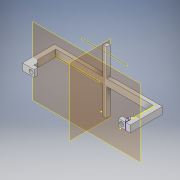
# Autodesk Inventor part: tec_holder_part2
Saved by Autodesk Inventor 2018 (Build 220112000, 112)
## iProperties
Created: 2018-02-10
Part Number: tec_holder_part2
Material: Generic
Document SubType Name: Modeling
Designer: Benedikt
Density: 1 g/cm^3
Appearance: Default
Author: Benedikt
## iProperties of the stored document tec_holder_part2_3DPrint.ipt
Created: 2018-02-10
Part Number: tec_holder_part2_3DPrint
Material: Generic
Document SubType Name: Modeling
Designer: Benedikt
Density: 1 g/cm^3
Appearance: Default
Author: Benedikt
Autodesk Inventor part; units mm, degrees
ref_plane "YZ Plane" through (0, 0, 0) normal (1, 0, 0) x (0, 1, 0)
ref_plane "XZ Plane" through (0, 0, 0) normal (0, 1, 0) x (-1, 0, 0)
ref_plane "XY Plane" through (0, 0, 0) normal (0, 0, 1) x (1, 0, 0)
ref_plane "Work Plane1" through (-37.0541, 3.9333, 19.6842) normal (0, 1, 0) x (-1, 0, 0)
sketch "Sketch1" plane through (-37.0541, 3.9333, 19.6842) normal (0, 1, 0) x (-1, 0, 0)
  point P0 (-37.0541, -19.6842)
ref_plane "Work Plane2" through (-37.0541, 26.9333, 19.6842) normal (0, 1, 0) x (-1, 0, 0)
sketch "Sketch2" plane through (-37.0541, 26.9333, 19.6842) normal (0, 1, 0) x (-1, 0, 0)
  line L0 (-16.9, -6.2922) -> (-16.9, -34.5181) construction
  line L1 (-18.4, -45.1) -> (-15.4, -45.1)
  line L2 (-15.4, 4.9) -> (-18.4, 4.9)
  line L3 (-15.4, -45.1) -> (-16.9, -20.1) construction
  line L4 (-17.065, -17.35) -> (-18.4, 4.9) construction
  line L5 (26.6, -17.35) -> (-15.4, -17.35)
  line L6 (-16.735, -17.35) -> (-17.065, -17.35)
  line L7 (-18.4, -17.35) -> (-60.4, -17.35)
  line L8 (-18.4, 4.9) -> (-18.4, -17.35)
  line L9 (-18.4, -22.85) -> (-18.4, -45.1)
  line L10 (-15.4, -45.1) -> (-15.4, -22.85)
  line L11 (-15.4, -17.35) -> (-15.4, 4.9)
  line L12 (-15.4, -22.85) -> (26.6, -22.85)
  line L13 (-18.4, -45.1) -> (-17.065, -22.85) construction
  line L14 (-16.9, -20.1) -> (-15.4, 4.9) construction
  line L15 (-60.4, -22.85) -> (-18.4, -22.85)
  line L16 (-17.065, -22.85) -> (-16.735, -22.85)
  line L17 (-60.4, -17.35) -> (-60.4, -22.85)
  line L18 (26.6, -17.35) -> (26.6, -22.85)
  point P0 (-37.0541, -19.6842)
  point P1 (22.6, -17.35)
  point P2 (-56.4, -22.85)
  dimension "d3" = 3
  dimension "d4" = 50
  dimension "d5" = 42
  dimension "d6" = 42
  constraints: 38 end point, 14 parallel, 4 horizontal, 3 perpendicular, 3 point on line, 2 vertical, 2 other
  measures "d3" distance of L2.end L2.start
  measures "d4" distance of L2.start L1.end
  measures "d5" distance between parallel lines of L9 L17
  measures "d6" distance between parallel lines of L18 L10
extrude "Extrusion2" add sketch "Sketch2" along normal blind 3
sketch "Sketch3" plane through (-37.0541, 26.9333, 19.6842) normal (0, -1, 0) x (1, 0, 0)
  line L0 (60.4, -22.85) -> (18.4, -22.85) projected
  line L1 (18.4, -17.35) -> (60.4, -17.35) projected
  line L2 (60.4, -22.85) -> (56.4, -22.85)
  line L3 (56.4, -22.85) -> (56.4, -17.35)
  line L4 (56.4, -17.35) -> (60.4, -17.35)
  line L5 (60.4, -17.35) -> (60.4, -22.85)
  line L6 (-26.6, -22.85) -> (-26.6, -17.35) projected
  line L7 (-26.6, -17.35) -> (15.4, -17.35) projected
  line L8 (-26.6, -22.85) -> (-22.6, -22.85)
  line L9 (-22.6, -22.85) -> (-22.6, -17.35)
  line L10 (-22.6, -17.35) -> (-26.6, -17.35)
  line L11 (-26.6, -17.35) -> (-26.6, -22.85)
  point P0 (37.0541, -19.6842)
  dimension "d9" = 4
  dimension "d10" = 4
  constraints: 16 end point, 4 parallel, 2 horizontal, 2 perpendicular, 2 point on line
  measures "d9" distance of L3.end L4.end
  measures "d10" distance of L10.end L9.end
extrude "Extrusion3" add sketch "Sketch3" along normal blind 23
sketch "Sketch4" plane through (19.3459, 26.9333, -3.1658) normal (-1, 0, 0) x (0, 0, 1)
  line L0 (5.5, -23) -> (0, -23) projected
  line L1 (5.5, 0) -> (5.5, -23) projected
  line L2 (0, -23) -> (5.5, -23)
  line L3 (5.5, -23) -> (5.5, -19)
  line L4 (5.5, -19) -> (0, -19)
  line L5 (0, -19) -> (0, -23)
  point P0 (3.1658, -26.9333)
  dimension "d13" = 4
  constraints: 8 end point, 2 parallel, 1 horizontal, 1 perpendicular, 1 point on line
  measures "d13" distance of L3.end L2.end
sketch "Sketch5" plane through (-18.6541, 29.9333, 2.3342) normal (0, 0, 1) x (1, 0, 0)
  line L0 (38, -3) -> (38, -26) projected
  line L1 (38, -26) -> (32.5, -26)
  line L2 (32.5, -26) -> (32.5, -23)
  line L3 (32.5, -23) -> (38, -17.8732)
  point P0 (18.6541, -29.9333)
  dimension "d14" = 5.5
  dimension "d15" = 3
  constraints: 6 end point, 1 horizontal, 1 perpendicular, 1 point on line
  measures "d14" distance of L0.end L1.end
  measures "d15" distance of L1.end L2.end
extrude "Extrusion4" add sketch "Sketch5" against normal up to surface (5.5 mm away)
ref_plane "Work Plane3" through (-20.1541, 26.9333, 2.3342) normal (1, 0, 0) x (0, 0, -1)
mirror "Mirror1" about plane through (-20.1541, 26.9333, 2.3342) normal (1, 0, 0) of "Extrusion4"
ref_plane "Work Plane4" through (-37.0541, 12.1833, 19.6842) normal (0, -1, 0) x (1, 0, 0)
sketch "Sketch6" plane through (-37.0541, 12.1833, 19.6842) normal (0, -1, 0) x (1, 0, 0)
  circle A0 centre (53.4, -20.1) radius 1.7 projected
  circle A1 centre (-19.6, -20.1) radius 1.7 projected
  line L0 (-16.8355, -21.7765) -> (-19.6696, -23.3324)
  line L1 (-19.6696, -23.3324) -> (-22.4342, -21.6559)
  line L2 (-22.4342, -21.6559) -> (-22.3645, -18.4234)
  line L3 (-22.3645, -18.4234) -> (-19.5303, -16.8676)
  line L4 (-19.5303, -16.8676) -> (-16.7658, -18.5441)
  line L5 (-16.7658, -18.5441) -> (-16.8355, -21.7765)
  line L6 (-19.6696, -23.3324) -> (-15.5487, -23.3324)
  line L7 (-15.5487, -23.3324) -> (-15.5487, -16.0828)
  line L8 (-15.5487, -16.0828) -> (-19.5303, -16.8676)
  point P0 (37.0541, -19.6842)
  dimension "d19" = 5.6
  constraints: 18 end point, 1 coincident, 1 horizontal, 1 perpendicular, 13 other
  measures "d19" distance between parallel lines of L1 L4
extrude "Extrusion5" cut sketch "Sketch6" along normal blind 5.25 contours A1 | L5 L4 L8 L7 L6 L0 | L0 L1 L2 L3 L4 L5
sketch "Sketch7" plane through (-37.0541, 3.9333, 19.6842) normal (0, -1, 0) x (1, 0, 0)
  circle A0 centre (-19.6, -20.1) radius 1.7 projected
  point P0 (37.0541, -19.6842)
extrude "Extrusion6" cut sketch "Sketch7" against normal blind 6.25
mirror "Mirror2" about plane through (-20.1541, 26.9333, 2.3342) normal (1, 0, 0) of "Extrusion5", "Extrusion6"
body "Solid2"
